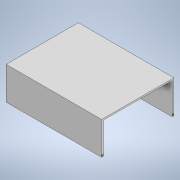
# Autodesk Inventor part: Powersupply_holder
Saved by Autodesk Inventor 2020 (Build 240168000, 168)
## iProperties
Created: 2020-05-27
Part Number: Powersupply_holder
Material: Generic
Document SubType Name: Modeling
Designer: Gebruiker
Density: 1 g/cm^3
Appearance: Default
Author: Gebruiker
Autodesk Inventor part; units mm, degrees
ref_plane "YZ Plane" through (0, 0, 0) normal (1, 0, 0) x (0, 1, 0)
ref_plane "XZ Plane" through (0, 0, 0) normal (0, 1, 0) x (-1, 0, 0)
ref_plane "XY Plane" through (0, 0, 0) normal (0, 0, 1) x (1, 0, 0)
sketch "Sketch1" plane through (0, 0, 0) normal (0, 0, 1) x (1, 0, 0)
  line L0 (0, 0) -> (160, 0)
  line L1 (160, 0) -> (160, 55)
  line L2 (160, 55) -> (0, 55)
  line L3 (0, 55) -> (0, 0)
  dimension "d0" = 160
  dimension "d1" = 55
  constraints: 8 end point, 2 parallel, 1 horizontal, 1 perpendicular
  measures "d0" distance of L2.end L1.end
  measures "d1" distance of L1.end L0.end
extrude "Extrusion1" add sketch "Sketch1" against normal blind 121
sketch "Sketch2" plane through (160, 0, 0) normal (1, 0, 0) x (0, 0, -1)
  line L0 (0, 55) -> (121, 55) construction
  line L1 (60.5, 55) -> (60.5, 0) construction
  line L2 (0, 0) -> (121, 0) construction
  line L3 (3, -0.4008) -> (118, -0.4008)
  line L4 (118, -0.4008) -> (118, 52.5992)
  line L5 (118, 52.5992) -> (3, 52.5992)
  line L6 (3, 52.5992) -> (3, -0.4008)
  point P0 (60.5, 27.5)
  dimension "d4" = 115
  dimension "d5" = 53
  constraints: 12 end point, 3 midpoint, 1 parallel, 1 perpendicular
  measures "d4" distance of L5.end L4.end
  measures "d5" distance of L4.end L3.end
extrude "Extrusion2" cut sketch "Sketch2" against normal blind 157
sketch "Sketch3" plane through (3, 0, 0) normal (1, 0, 0) x (0, 0, -1)
  line L0 (3, 52.5992) -> (118, 52.5992) construction
  line L1 (60.5, 52.5992) -> (60.5, 0) construction
  line L2 (118, 0) -> (3, 0) construction
  line L3 (3, 0) -> (3, 52.5992) construction
  line L4 (3, 26.2996) -> (118, 26.2996) construction
  line L5 (118, 52.5992) -> (118, 0) construction
  line L6 (15.3897, 46.9324) -> (11.2242, 41.2554)
  line L7 (18.2655, 41.2554) -> (15.3897, 46.9324)
  line L8 (11.2242, 41.2554) -> (18.2655, 41.2554)
  line L9 (19.3897, 46.9324) -> (22.2655, 41.2554)
  line L10 (22.2655, 41.2554) -> (26.431, 46.9324)
  line L11 (26.431, 46.9324) -> (19.3897, 46.9324)
  line L12 (30.431, 47.8673) -> (26.8829, 41.4481)
  line L13 (34.2174, 41.4481) -> (30.431, 47.8673)
  line L14 (26.8829, 41.4481) -> (34.2174, 41.4481)
  line L15 (46.7018, 47.8787) -> (42.5363, 41.455)
  line L16 (50.1923, 41.455) -> (46.7018, 47.8787)
  line L17 (42.5363, 41.455) -> (50.1923, 41.455)
  line L18 (34.431, 47.8477) -> (38.5363, 41.424)
  line L19 (38.5363, 41.424) -> (42.7018, 47.8477)
  line L20 (42.7018, 47.8477) -> (34.431, 47.8477)
  line L21 (3.7337, 47.9702) -> (7.2242, 41.5465)
  line L22 (7.2242, 41.5465) -> (11.3897, 47.9702)
  line L23 (11.3897, 47.9702) -> (3.7337, 47.9702)
  line L24 (54.1923, 41.2928) -> (58.3578, 47.7164)
  line L25 (58.3578, 47.7164) -> (50.7018, 47.7164)
  line L26 (50.7018, 47.7164) -> (54.1923, 41.2928)
  line L27 (3, 52.5992) -> (60.5, 26.2996) construction
  line L28 (60.5, 52.5992) -> (3, 26.2996) construction
  line L29 (3, 39.4494) -> (60.5, 39.4494) construction
  line L30 (15.3897, 31.9665) -> (11.2242, 37.6435)
  line L31 (18.2655, 37.6435) -> (15.3897, 31.9665)
  line L32 (11.2242, 37.6435) -> (18.2655, 37.6435)
  line L33 (19.3897, 31.9665) -> (22.2655, 37.6435)
  line L34 (22.2655, 37.6435) -> (26.431, 31.9665)
  line L35 (26.431, 31.9665) -> (19.3897, 31.9665)
  line L36 (34.2174, 37.4507) -> (30.431, 31.0315)
  line L37 (30.431, 31.0315) -> (26.8829, 37.4507)
  line L38 (26.8829, 37.4507) -> (34.2174, 37.4507)
  line L39 (50.1923, 37.4439) -> (46.7018, 31.0202)
  line L40 (46.7018, 31.0202) -> (42.5363, 37.4439)
  line L41 (42.5363, 37.4439) -> (50.1923, 37.4439)
  line L42 (38.5363, 37.4748) -> (42.7018, 31.0512)
  line L43 (42.7018, 31.0512) -> (34.431, 31.0512)
  line L44 (34.431, 31.0512) -> (38.5363, 37.4748)
  line L45 (7.2242, 37.3524) -> (11.3897, 30.9287)
  line L46 (11.3897, 30.9287) -> (3.7337, 30.9287)
  line L47 (3.7337, 30.9287) -> (7.2242, 37.3524)
  line L48 (54.1923, 37.6061) -> (58.3578, 31.1825)
  line L49 (58.3578, 31.1825) -> (50.7018, 31.1825)
  line L50 (50.7018, 31.1825) -> (54.1923, 37.6061)
  line L51 (118, 26.2996) -> (3, 26.2996) construction
  line L52 (105.6103, 46.9324) -> (109.7758, 41.2554)
  line L53 (102.7345, 41.2554) -> (105.6103, 46.9324)
  line L54 (109.7758, 41.2554) -> (102.7345, 41.2554)
  line L55 (101.6103, 46.9324) -> (98.7345, 41.2554)
  line L56 (98.7345, 41.2554) -> (94.569, 46.9324)
  line L57 (94.569, 46.9324) -> (101.6103, 46.9324)
  line L58 (86.7826, 41.4481) -> (90.569, 47.8673)
  line L59 (90.569, 47.8673) -> (94.1171, 41.4481)
  line L60 (94.1171, 41.4481) -> (86.7826, 41.4481)
  line L61 (70.8077, 41.455) -> (74.2982, 47.8787)
  line L62 (74.2982, 47.8787) -> (78.4637, 41.455)
  line L63 (78.4637, 41.455) -> (70.8077, 41.455)
  line L64 (82.4637, 41.424) -> (78.2982, 47.8477)
  line L65 (78.2982, 47.8477) -> (86.569, 47.8477)
  line L66 (86.569, 47.8477) -> (82.4637, 41.424)
  line L67 (113.7758, 41.5465) -> (109.6103, 47.9702)
  line L68 (109.6103, 47.9702) -> (117.2663, 47.9702)
  line L69 (117.2663, 47.9702) -> (113.7758, 41.5465)
  line L70 (66.8077, 41.2928) -> (62.6422, 47.7164)
  line L71 (62.6422, 47.7164) -> (70.2982, 47.7164)
  line L72 (70.2982, 47.7164) -> (66.8077, 41.2928)
  line L73 (113.7758, 37.3524) -> (109.6103, 30.9287)
  line L74 (109.6103, 30.9287) -> (117.2663, 30.9287)
  line L75 (117.2663, 30.9287) -> (113.7758, 37.3524)
  line L76 (105.6103, 31.9665) -> (109.7758, 37.6435)
  line L77 (102.7345, 37.6435) -> (105.6103, 31.9665)
  line L78 (109.7758, 37.6435) -> (102.7345, 37.6435)
  line L79 (101.6103, 31.9665) -> (98.7345, 37.6435)
  line L80 (98.7345, 37.6435) -> (94.569, 31.9665)
  line L81 (94.569, 31.9665) -> (101.6103, 31.9665)
  line L82 (90.569, 31.0315) -> (94.1171, 37.4507)
  line L83 (94.1171, 37.4507) -> (86.7826, 37.4507)
  line L84 (86.7826, 37.4507) -> (90.569, 31.0315)
  line L85 (86.569, 31.0512) -> (82.4637, 37.4748)
  line L86 (78.2982, 31.0512) -> (86.569, 31.0512)
  line L87 (82.4637, 37.4748) -> (78.2982, 31.0512)
  line L88 (74.2982, 31.0202) -> (78.4637, 37.4439)
  line L89 (78.4637, 37.4439) -> (70.8077, 37.4439)
  line L90 (70.8077, 37.4439) -> (74.2982, 31.0202)
  line L91 (70.2982, 31.1825) -> (66.8077, 37.6061)
  line L92 (62.6422, 31.1825) -> (70.2982, 31.1825)
  line L93 (66.8077, 37.6061) -> (62.6422, 31.1825)
  line L94 (15.3897, 5.6669) -> (11.2242, 11.3439)
  line L95 (18.2655, 11.3439) -> (15.3897, 5.6669)
  line L96 (11.2242, 11.3439) -> (18.2655, 11.3439)
  line L97 (19.3897, 5.6669) -> (22.2655, 11.3439)
  line L98 (22.2655, 11.3439) -> (26.431, 5.6669)
  line L99 (26.431, 5.6669) -> (19.3897, 5.6669)
  line L100 (34.2174, 11.1511) -> (30.431, 4.7319)
  line L101 (30.431, 4.7319) -> (26.8829, 11.1511)
  line L102 (26.8829, 11.1511) -> (34.2174, 11.1511)
  line L103 (50.1923, 11.1442) -> (46.7018, 4.7206)
  line L104 (46.7018, 4.7206) -> (42.5363, 11.1442)
  line L105 (42.5363, 11.1442) -> (50.1923, 11.1442)
  line L106 (38.5363, 11.1752) -> (42.7018, 4.7516)
  line L107 (42.7018, 4.7516) -> (34.431, 4.7516)
  line L108 (34.431, 4.7516) -> (38.5363, 11.1752)
  line L109 (7.2242, 11.0527) -> (11.3897, 4.6291)
  line L110 (11.3897, 4.6291) -> (3.7337, 4.6291)
  line L111 (3.7337, 4.6291) -> (7.2242, 11.0527)
  line L112 (54.1923, 11.3065) -> (58.3578, 4.8828)
  line L113 (58.3578, 4.8828) -> (50.7018, 4.8828)
  line L114 (50.7018, 4.8828) -> (54.1923, 11.3065)
  line L115 (7.2242, 15.2469) -> (11.3897, 21.6705)
  line L116 (11.3897, 21.6705) -> (3.7337, 21.6705)
  line L117 (3.7337, 21.6705) -> (7.2242, 15.2469)
  line L118 (15.3897, 20.6327) -> (11.2242, 14.9558)
  line L119 (18.2655, 14.9558) -> (15.3897, 20.6327)
  line L120 (11.2242, 14.9558) -> (18.2655, 14.9558)
  line L121 (19.3897, 20.6327) -> (22.2655, 14.9558)
  line L122 (22.2655, 14.9558) -> (26.431, 20.6327)
  line L123 (26.431, 20.6327) -> (19.3897, 20.6327)
  line L124 (30.431, 21.5677) -> (26.8829, 15.1485)
  line L125 (26.8829, 15.1485) -> (34.2174, 15.1485)
  line L126 (34.2174, 15.1485) -> (30.431, 21.5677)
  line L127 (34.431, 21.5481) -> (38.5363, 15.1244)
  line L128 (42.7018, 21.5481) -> (34.431, 21.5481)
  line L129 (38.5363, 15.1244) -> (42.7018, 21.5481)
  line L130 (46.7018, 21.579) -> (42.5363, 15.1554)
  line L131 (42.5363, 15.1554) -> (50.1923, 15.1554)
  line L132 (50.1923, 15.1554) -> (46.7018, 21.579)
  line L133 (50.7018, 21.4168) -> (54.1923, 14.9931)
  line L134 (58.3578, 21.4168) -> (50.7018, 21.4168)
  line L135 (54.1923, 14.9931) -> (58.3578, 21.4168)
  line L136 (113.7758, 11.0527) -> (109.6103, 4.6291)
  line L137 (109.6103, 4.6291) -> (117.2663, 4.6291)
  line L138 (117.2663, 4.6291) -> (113.7758, 11.0527)
  line L139 (105.6103, 5.6669) -> (109.7758, 11.3439)
  line L140 (102.7345, 11.3439) -> (105.6103, 5.6669)
  line L141 (109.7758, 11.3439) -> (102.7345, 11.3439)
  line L142 (101.6103, 5.6669) -> (98.7345, 11.3439)
  line L143 (94.569, 5.6669) -> (101.6103, 5.6669)
  line L144 (98.7345, 11.3439) -> (94.569, 5.6669)
  line L145 (90.569, 4.7319) -> (94.1171, 11.1511)
  line L146 (86.7826, 11.1511) -> (90.569, 4.7319)
  line L147 (94.1171, 11.1511) -> (86.7826, 11.1511)
  line L148 (86.569, 4.7516) -> (82.4637, 11.1752)
  line L149 (78.2982, 4.7516) -> (86.569, 4.7516)
  line L150 (82.4637, 11.1752) -> (78.2982, 4.7516)
  line L151 (74.2982, 4.7206) -> (78.4637, 11.1442)
  line L152 (70.8077, 11.1442) -> (74.2982, 4.7206)
  line L153 (78.4637, 11.1442) -> (70.8077, 11.1442)
  line L154 (70.2982, 4.8828) -> (66.8077, 11.3065)
  line L155 (62.6422, 4.8828) -> (70.2982, 4.8828)
  line L156 (66.8077, 11.3065) -> (62.6422, 4.8828)
  line L157 (70.2982, 21.4168) -> (66.8077, 14.9931)
  line L158 (66.8077, 14.9931) -> (62.6422, 21.4168)
  line L159 (62.6422, 21.4168) -> (70.2982, 21.4168)
  line L160 (70.8077, 15.1554) -> (74.2982, 21.579)
  line L161 (78.4637, 15.1554) -> (70.8077, 15.1554)
  line L162 (74.2982, 21.579) -> (78.4637, 15.1554)
  line L163 (82.4637, 15.1244) -> (78.2982, 21.5481)
  line L164 (86.569, 21.5481) -> (82.4637, 15.1244)
  line L165 (78.2982, 21.5481) -> (86.569, 21.5481)
  line L166 (86.7826, 15.1485) -> (90.569, 21.5677)
  line L167 (94.1171, 15.1485) -> (86.7826, 15.1485)
  line L168 (90.569, 21.5677) -> (94.1171, 15.1485)
  line L169 (98.7345, 14.9558) -> (94.569, 20.6327)
  line L170 (101.6103, 20.6327) -> (98.7345, 14.9558)
  line L171 (94.569, 20.6327) -> (101.6103, 20.6327)
  line L172 (102.7345, 14.9558) -> (105.6103, 20.6327)
  line L173 (109.7758, 14.9558) -> (102.7345, 14.9558)
  line L174 (105.6103, 20.6327) -> (109.7758, 14.9558)
  line L175 (113.7758, 15.2469) -> (109.6103, 21.6705)
  line L176 (117.2663, 21.6705) -> (113.7758, 15.2469)
  line L177 (109.6103, 21.6705) -> (117.2663, 21.6705)
  circle A0 centre (60.5, 13.1498) radius 3.5
  circle A1 centre (60.5, 39.4494) radius 3.5
  line L178 (3, 26.2996) -> (60.5, 0) construction
  line L179 (3, 0) -> (3, 52.5992) construction
  line L180 (60.5, 26.2996) -> (3, 0) construction
  line L181 (3, 0) -> (3, 13.1498) construction
  line L182 (3, 13.1498) -> (118, 13.1498) construction
  point P0 (0, 0)
  dimension "d9" = 4
  dimension "d10" = 4
  dimension "d11" = 4
  dimension "d12" = 4
  dimension "d14" = 4
  dimension "d17" = 7
  dimension "d18" = 7
  constraints: 356 end point, 149 symmetric about line, 6 midpoint, 5 equal length, 5 point on line, 4 horizontal, 2 centre point, 2 perpendicular, 1 parallel
  measures "d9" distance of L9.start L6.start
  measures "d10" horizontal distance of L13.end L10.end
  measures "d11" horizontal distance of L6.start L22.end
  measures "d12" horizontal distance of L20.end L13.end
  measures "d14" horizontal distance of L25.end L16.end
  measures "d17" diameter of A0
  measures "d18" diameter of A1
extrude "Extrusion3" cut sketch "Sketch3" against normal blind 5 contours L7 L8 L6 | L11 L10 L9 | L13 L14 L12 | L16 L17 L15 | L20 L19 L18 | L23 L22 L21 | L26 L25 L24 | L30 L32 L31 | L33 L34 L35 | L36 L37 L38 | L39 L40 L41 | L42 L43 L44 | L45 L46 L47 | L48 L49 L50 | L52 L54 L53 | L55 L56 L57 | L58 L59 L60 | L61 L62 L63 | L64 L65 L66 | L67 L68 L69 | L70 L71 L72 | L75 L74 L73 | L77 L78 L76 | L81 L80 L79 | L84 L83 L82 | L86 L87 L85 | L90 L89 L88 | L92 L93 L91 | L94 L96 L95 | L97 L98 L99 | L100 L101 L102 | L103 L104 L105 | L106 L107 L108 | L109 L110 L111 | L112 L113 L114 | L117 L116 L115 | L119 L120 L118 | L123 L122 L121 | L126 L125 L124 | L128 L129 L127 | L132 L131 L130 | L134 L135 L133 | L138 L137 L136 | L140 L141 L139 | L143 L144 L142 | L146 L147 L145 | L149 L150 L148 | L152 L153 L151 | L155 L156 L154 | L157 L158 L159 | L160 L162 L161 | L163 L165 L164 | L166 L168 L167 | L169 L171 L170 | L172 L174 L173 | L175 L177 L176
extrude "Extrusion4" cut sketch "Sketch3" against normal blind 5 contours A0 | A1
sketch "Sketch4" plane through (160, 0, 0) normal (1, 0, 0) x (0, 0, -1)
  line L0 (0, 0) -> (0, 55) construction
  line L1 (3, 0) -> (3, 52.5992) construction
  line L2 (0, 3.5046) -> (3, 0) construction
  line L3 (3, 0) -> (3, 3.5046) construction
  line L4 (0, 0) -> (3, 3.5046) construction
  line L5 (1.1, -3.5) -> (1.9, -3.5) construction
  line L6 (1.9, -3.5) -> (1.9, 3.5)
  line L7 (1.9, 3.5) -> (1.1, 3.5)
  line L8 (1.1, 3.5) -> (1.1, -3.5)
  line L9 (0, 0) -> (121, 0) construction
  line L10 (1.1, -3.5) -> (1.9, 3.5) construction
  line L11 (1.9, -3.5) -> (1.1, 3.5) construction
  line L12 (0.45, 2.1) -> (2.55, 2.1)
  line L13 (2.55, 2.1) -> (2.55, 3.5)
  line L14 (2.55, 3.5) -> (0.45, 3.5)
  line L15 (0.45, 3.5) -> (0.45, 2.1)
  line L16 (0.45, 2.1) -> (2.55, 3.5) construction
  line L17 (2.55, 2.1) -> (0.45, 3.5) construction
  line L18 (1.1, 0) -> (1.9, 0)
  point P0 (1.5, 0)
  point P1 (1.5, 2.8)
  point P2 (1.9, 2.1)
  point P3 (1.1, 2.1)
  dimension "d21" = 0.8
  dimension "d22" = 7
  dimension "d23" = 2.1
  dimension "d24" = 1.4
  constraints: 32 end point, 6 midpoint, 5 point on line, 4 parallel, 2 horizontal, 2 perpendicular, 1 collinear
  measures "d21" distance of L7.end L6.end
  measures "d22" distance of L6.end L5.end
  measures "d23" distance of L14.end L13.end
  measures "d24" distance of L13.end L12.end
extrude "Extrusion5" cut sketch "Sketch4" against normal blind 160
sketch "Sketch5" plane through (160, 0, 0) normal (1, 0, 0) x (0, 0, -1)
  line L0 (119.1, -3.5) -> (119.9, -3.5)
  line L1 (119.9, -3.5) -> (119.9, 3.5)
  line L2 (119.9, 3.5) -> (119.1, 3.5)
  line L3 (119.1, 3.5) -> (119.1, -3.5)
  line L4 (118, 0) -> (121, 0) projected
  line L5 (119.1, -3.5) -> (119.9, 3.5) construction
  line L6 (119.9, -3.5) -> (119.1, 3.5) construction
  line L7 (118.45, 2.1) -> (120.55, 2.1)
  line L8 (120.55, 2.1) -> (120.55, 3.5)
  line L9 (120.55, 3.5) -> (118.45, 3.5)
  line L10 (118.45, 3.5) -> (118.45, 2.1)
  line L11 (118.45, 2.1) -> (120.55, 3.5) construction
  line L12 (120.55, 2.1) -> (118.45, 3.5) construction
  line L13 (119.1, 0) -> (119.9, 0)
  point P0 (0, 0)
  point P1 (119.5, 0)
  point P2 (119.5, 2.8)
  point P3 (119.1, 2.1)
  point P4 (119.9, 2.1)
  dimension "d27" = 0.8
  dimension "d28" = 7
  dimension "d29" = 2.1
  dimension "d30" = 1.4
  constraints: 26 end point, 7 midpoint, 4 parallel, 2 horizontal, 2 perpendicular, 2 point on line, 1 collinear
  measures "d27" distance of L2.end L1.end
  measures "d28" distance of L1.end L0.end
  measures "d29" distance of L9.end L8.end
  measures "d30" distance of L8.end L7.end
extrude "Extrusion6" cut sketch "Sketch5" against normal blind 160 contours L3 L7 L1 L4 | L7 L10 L9 L3 | L3 L2 L1 L7 | L1 L9 L8 L7
body "Solid1"
